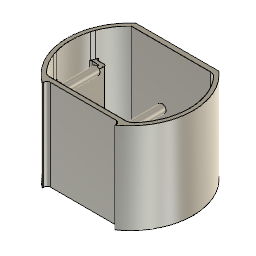
MotorControllerMount (Autodesk Fusion 360 design; units mm, degrees)
Autodesk Fusion 360 part; units mm, degrees
sketch "Sketch1" plane through (0, 0, 0) normal (0, 0, 1) x (1, 0, 0)
  circle A0 centre (0, 0) radius 35.814
  circle A1 centre (0, 0) radius 38.1
  line L0 (-25, -25.6445) -> (25, -25.6445)
  line L1 (-25, 25.6445) -> (-25, -25.6445)
  line L2 (-25, 25.6445) -> (28.1774, 25.6445)
  line L3 (-25, 25.6445) -> (-28.1774, 25.6445)
  line L4 (-22, -31.1064) -> (-22, -28.2603)
  line L5 (-22, -28.2603) -> (22, -28.2603)
  line L6 (22, -31.1064) -> (22, -28.2603)
  line L7 (-25.1217, 28.6445) -> (25.1217, 28.6445)
  line L8 (12.5, 25.6445) -> (-12.5, 25.6445)
  line L9 (-12.5, 25.6445) -> (-12.5, 21.6445)
  line L10 (-12.5, 21.6445) -> (12.5, 21.6445)
  line L11 (12.5, 21.6445) -> (12.5, 25.6445)
  line L12 (14.5, 25.6445) -> (-14.5, 25.6445)
  line L13 (-14.5, 25.6445) -> (-14.5, 19.6445)
  line L14 (-14.5, 19.6445) -> (14.5, 19.6445)
  line L15 (14.5, 19.6445) -> (14.5, 25.6445)
  line L16 (0, 21.6445) -> (0, 25.6445)
  line L17 (0, 25.6445) -> (0, 0) construction
  line L18 (34.2402, 10.5) -> (29, 10.5)
  line L19 (29, 10.5) -> (29, -10.5)
  line L20 (29, -10.5) -> (34.2402, -10.5)
  line L21 (33.5618, -12.5) -> (27, -12.5)
  line L22 (27, -12.5) -> (27, 12.5)
  line L23 (27, 12.5) -> (33.5618, 12.5)
  line L24 (27, 0) -> (0, 0) construction
  line L25 (-27, -12.5) -> (-27, 12.5)
  line L26 (-29, 10.5) -> (-29, -10.5)
  line L27 (-34.2402, 10.5) -> (-29, 10.5)
  line L28 (-27, 12.5) -> (-33.5618, 12.5)
  line L29 (-29, -10.5) -> (-34.2402, -10.5)
  line L30 (-33.5618, -12.5) -> (-27, -12.5)
  dimension "d1" = 76.2
  dimension "d3" = 50
  dimension "d15" = 3
  dimension "d16" = 3
  dimension "d24" = 2
  dimension "d25" = 2
  dimension "d26" = 2
  dimension "d27" = 25
  dimension "d28" = 6
  dimension "d37" = 2
  dimension "d38" = 25
  dimension "d39" = 2
  dimension "d40" = 2
  dimension "d41" = 2
  dimension "d60" = 71.628
  constraint coincident A0.centre A1.centre
  constraint coincident A0 L0.start
  constraint coincident A0 L0.end
  constraint horizontal L0
  constraint coincident A0 L1.start
  constraint perpendicular L0 L1
  constraint coincident A1 L2.end
  constraint perpendicular L1 L2
  constraint coincident A1 L3.end
  constraint perpendicular L1 L3
  constraint coincident A1 L4.start
  constraint vertical L4
  constraint perpendicular L4 L5
  constraint coincident A1 L6.start
  constraint perpendicular L5 L6
  constraint coincident A1 L7.start
  constraint coincident A1 L7.end
  constraint perpendicular L6 L7
  constraint coincident A0 L5.end
  constraint horizontal L8
  constraint vertical L9
  constraint horizontal L10
  constraint vertical L11
  constraint coincident L2 L8.start
  constraint horizontal L12
  constraint vertical L13
  constraint horizontal L14
  constraint vertical L15
  constraint coincident L2 L12.start
  constraint midpoint L10 L16.start
  constraint perpendicular L8 L16
  constraint coincident L2 L16.end
  constraint perpendicular L8 L17
  constraint coincident A0 L18.start
  constraint horizontal L18
  constraint perpendicular L18 L19
  constraint coincident A0 L20.end
  constraint perpendicular L19 L20
  constraint coincident A0 L21.start
  constraint parallel L20 L21
  constraint perpendicular L21 L22
  constraint coincident A0 L23.end
  constraint perpendicular L22 L23
  constraint coincident L22 L24.start
  constraint midpoint L22 L24.start
  constraint perpendicular L17 L24
  constraint symmetric L17 L18.start L27.start
  constraint symmetric L17 L18.end L26.start
  constraint symmetric L17 L19.end L26.end
  constraint symmetric L17 L20.end L29.end
  constraint symmetric L17 L21.start L30.start
  constraint symmetric L17 L21.end L25.start
  constraint symmetric L17 L22.end L25.end
  constraint symmetric L17 L23.end L28.end
  constraint coincident A0 L4.end
  measures "d1" diameter of A1
  measures "d3" distance of L0.start L0.end
  measures "d15" distance of L2 L7
  measures "d16" horizontal distance of L0.end L6.start
  measures "d24" distance of L10 L14
  measures "d25" distance of L9 L13
  measures "d26" distance of L11 L15
  measures "d27" distance of L9.end L10.end
  measures "d28" distance of L12.start L14.end
  measures "d37" distance of L19 L22
  measures "d38" distance of L21.end L22.end
  measures "d39" distance of L18 L23
  measures "d40" distance of L20 L21
  measures "d41" distance of L0.end L22
  measures "d60" diameter of A0
extrude "Extrude1" add sketch "Sketch1" along normal blind 55 contours A0 A1 L2 L6 | A0 L18 L19 L20 L21 L22 L23 | A0 L2 L7 L8 L12 | A0 A1 L2 L7 | A0 L0 L5 | A0 A1 L3 L4 | A0 A1 L3 L7 | A0 L25 L26 L27 L28 L29 L30
sketch "Sketch3" plane through (0, -25.6445, 0) normal (0, 1, 0) x (-1, 0, 0)
  line L0 (-25, 0) -> (25, 0)
  line L1 (25, 0) -> (25, 55)
  line L2 (25, 55) -> (-25, 55)
  line L3 (-25, 55) -> (-25, 0)
  line L4 (0, 0) -> (0, 27.5) construction
  line L5 (-25, 27.5) -> (0, 27.5) construction
  line L6 (0, 27.5) -> (-19.997, 7.503) construction
  circle A0 centre (-19.997, 7.503) radius 1.5
  circle A1 centre (-19.997, 7.503) radius 2.5
  circle A2 centre (19.997, 7.503) radius 2.5
  circle A3 centre (19.997, 7.503) radius 1.5
  circle A4 centre (19.997, 47.497) radius 2.5
  circle A5 centre (19.997, 47.497) radius 1.5
  circle A6 centre (-19.997, 47.497) radius 2.5
  circle A7 centre (-19.997, 47.497) radius 1.5
  dimension "d7" = 45
  dimension "d8" = 28.28
  dimension "d9" = 3
  dimension "d10" = 5
  dimension "d12" = 360
  constraint coincident L4.start origin
  constraint perpendicular L0 L4
  constraint midpoint L3 L5.start
  constraint perpendicular L3 L5
  constraint coincident L6.end A0.centre
  constraint concentric A0 A1
  measures "d7" angle of L5 L6
  measures "d8" distance of L4.end L6.end
  measures "d9" diameter of A0
  measures "d10" diameter of A1
extrude "Extrude2" add sketch "Sketch3" along normal blind 25 contours A1 | A2 | A4 | A6
fillet "Fillet1" radius 2 2 edges at (22, -28.2603, 27.5) (-22, -28.2603, 27.5)
fillet "Fillet2" radius 5 4 edges at (25, -25.6445, 27.5) (25, -25.6445, 27.5) (25, 25.6445, 27.5) (25, 25.6445, 27.5)
extrude "Extrude3" cut sketch "Sketch1" along normal blind 15 contours A0 L18 L19 L20 L21 L22 L23 | L2 L9 L10 L11 L12 L13 L14 L15 | A0 L25 L26 L27 L28 L29 L30
sketch "Sketch5" plane through (0, 0, 55) normal (0, 0, 1) x (-1, 0, 0)
  arc A0 (34.2402, -10.5) -> (34.2402, 10.5) centre (0, 0) ccw
  line L0 (34.2402, -10.5) -> (29, -10.5)
  line L1 (29, -10.5) -> (29, 10.5)
  line L2 (29, 10.5) -> (34.2402, 10.5)
  line L3 (-22.8759, 25.6445) -> (25, 25.6445)
  arc A1 (33.5618, 12.5) -> (25, 25.6445) centre (0, 0) ccw
  line L4 (33.5618, 12.5) -> (27, 12.5)
  line L5 (27, 12.5) -> (27, -12.5)
  line L6 (27, -12.5) -> (33.5618, -12.5)
  arc A2 (25, -25.6445) -> (33.5618, -12.5) centre (0, 0) ccw
  line L7 (25, -25.6445) -> (-22.8759, -25.6445)
  arc A3 (-26.5878, -23.9944) -> (-22.8759, -25.6445) centre (-22.8759, -20.6445) ccw
  arc A4 (-33.5618, -12.5) -> (-26.5878, -23.9944) centre (0, 0) ccw
  line L8 (-33.5618, -12.5) -> (-27, -12.5)
  line L9 (-27, -12.5) -> (-27, 12.5)
  line L10 (-27, 12.5) -> (-33.5618, 12.5)
  arc A5 (-26.5878, 23.9944) -> (-33.5618, 12.5) centre (0, 0) ccw
  arc A6 (-22.8759, 25.6445) -> (-26.5878, 23.9944) centre (-22.8759, 20.6445) ccw
  line L11 (-34.2402, 10.5) -> (-29, 10.5)
  line L12 (-29, 10.5) -> (-29, -10.5)
  line L13 (-29, -10.5) -> (-34.2402, -10.5)
  arc A7 (-34.2402, 10.5) -> (-34.2402, -10.5) centre (0, 0) ccw
  line L14 (22, 31.1064) -> (22, 30.2603)
  arc A8 (20, 28.2603) -> (22, 30.2603) centre (20, 30.2603) ccw
  line L15 (20, 28.2603) -> (-20, 28.2603)
  arc A9 (-22, 30.2603) -> (-20, 28.2603) centre (-20, 30.2603) ccw
  line L16 (-22, 30.2603) -> (-22, 31.1064)
  arc A10 (-22, 31.1064) -> (-25.1217, -28.6445) centre (0, 0) ccw
  line L17 (-25.1217, -28.6445) -> (25.1217, -28.6445)
  arc A11 (25.1217, -28.6445) -> (22, 31.1064) centre (0, 0) ccw
  line L18 (-33.5618, -12.5) -> (-34.2402, -10.5)
  line L19 (-34.2402, 10.5) -> (-33.5618, 12.5)
  line L20 (34.2402, 10.5) -> (33.5618, 12.5)
  line L21 (34.2402, -10.5) -> (33.5618, -12.5)
  constraint coincident A4.start L8.start
  constraint coincident L13.end A7.end
  constraint coincident L11.start A7.start
  constraint coincident L10.end A5.end
  constraint coincident A0.end L2.end
  constraint coincident A1.start L4.start
  constraint coincident A0.start L0.start
  constraint coincident L6.end A2.end
extrude "Extrude5" cut sketch "Sketch5" against normal blind 15 contours L0 L1 L2 L4 L5 L6 L20 L21 | L8 L9 L10 L11 L12 L13 L18 L19
fillet "Fillet6" radius 5 1 edges at (-25, -25.6445, 27.5)
fillet "Fillet7" radius 1 15 edges at (27, 12.5, 27.5) (27, -12.5, 27.5) (33.5618, -12.5, 27.5) (34.2402, 10.5, 27.5) (33.5618, 12.5, 27.5) (-27, 12.5, 27.5) (-27, -12.5, 27.5) (-34.2402, -10.5, 27.5) (-29, -10.5, 27.5) (-29, 10.5, 27.5) (-33.5618, 12.5, 27.5) (-33.5618, -12.5, 27.5) (29, -10.5, 27.5) (29, 10.5, 27.5) (34.2402, -10.5, 27.5)
fillet "Fillet8" radius 1 1 edges at (-34.2402, 10.5, 27.5)
equation "d8 = 20 * 1.414 mm"
named bodies: "MotorControllerMount"
